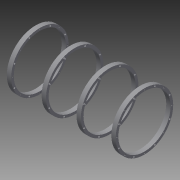
# Autodesk Inventor part: Part1
Saved by Autodesk Inventor 2015 (Build 190159000, 159)
## iProperties
Created: 2015-09-23
Part Number: Part1
Material: Generic
Document SubType Name: Modeling
Designer: Stefania
Density: 1 g/cm^3
Appearance: Default
Author: Stefania
Autodesk Inventor part; units mm, degrees
ref_plane "YZ Plane" through (0, 0, 0) normal (1, 0, 0) x (0, 1, 0)
ref_plane "XZ Plane" through (0, 0, 0) normal (0, 1, 0) x (-1, 0, 0)
ref_plane "Work Plane1" through (0, 0, 50.8) normal (0, 0, 1) x (1, 0, 0)
sketch "Sketch1" plane through (0, 0, 50.8) normal (0, 0, 1) x (1, 0, 0)
  circle A0 centre (0, 0) radius 76.2
  circle A1 centre (0, 0) radius 83.82
  dimension "d1" = 152.4
  dimension "d2" = 7.62
  constraints: 2 centre point, 1 coincident
  measures "d1" diameter of A0
  measures "d2" radial gap between concentric circles of A0 A1
extrude "Extrusion1" add sketch "Sketch1" along normal mid plane 12.7
pattern_linear "Rectangular Pattern1" count 3 spacing 101.6 along (0, 0, -1) count 2 spacing 101.6 along (0, 0, 1) of "Extrusion1"
sketch "Sketch2" plane through (0, 0, 158.75) normal (0, 0, 1) x (1, 0, 0)
  circle A0 centre (30.6185, 73.9196) radius 2.413
  circle A1 centre (-30.6185, 73.9196) radius 2.413
  circle A2 centre (-73.9196, 30.6185) radius 2.413
  circle A3 centre (-73.9196, -30.6185) radius 2.413
  circle A4 centre (-30.6185, -73.9196) radius 2.413
  circle A5 centre (30.6185, -73.9196) radius 2.413
  circle A6 centre (73.9196, -30.6185) radius 2.413
  circle A7 centre (73.9196, 30.6185) radius 2.413
  point P0 (0, 0)
  dimension "d16" = 4.826
  dimension "d19" = 360
  constraints: 8 centre point, 18 other
  measures "d16" diameter of A0
extrude "Extrusion2" cut sketch "Sketch2" against normal up to surface (12.7 mm away)
pattern_linear "Rectangular Pattern2" count 4 spacing 101.6 along (0, 0, -1) of "Extrusion2"
sketch "Sketch3" plane through (0, 0, 158.75) normal (0, 0, 1) x (1, 0, 0)
  circle A0 centre (0, 80.01) radius 1.7526
  circle A1 centre (-56.5756, 56.5756) radius 1.7526
  circle A2 centre (-80.01, 0) radius 1.7526
  circle A3 centre (-56.5756, -56.5756) radius 1.7526
  circle A4 centre (0, -80.01) radius 1.7526
  circle A5 centre (56.5756, -56.5756) radius 1.7526
  circle A6 centre (80.01, 0) radius 1.7526
  circle A7 centre (56.5756, 56.5756) radius 1.7526
  point P0 (0, 0)
  dimension "d26" = 3.5052
  dimension "d29" = 360
  constraints: 8 centre point, 18 other
  measures "d26" diameter of A0
extrude "Extrusion3" cut sketch "Sketch3" against normal up to surface (12.7 mm away)
pattern_linear "Rectangular Pattern4" count 2 spacing 304.8 along (0, 0, -1) of "Extrusion3"
thread "Thread1" size "6-32 UNC" class "2B" standard "ANSI Unified Screw Threads" full length
thread "Thread2" size "6-32 UNC" class "2B" standard "ANSI Unified Screw Threads" full length
thread "Thread3" size "6-32 UNC" class "2B" standard "ANSI Unified Screw Threads" full length
thread "Thread4" size "6-32 UNC" class "2B" standard "ANSI Unified Screw Threads" full length
thread "Thread5" size "6-32 UNC" class "2B" standard "ANSI Unified Screw Threads" full length
thread "Thread6" size "6-32 UNC" class "2B" standard "ANSI Unified Screw Threads" full length
thread "Thread7" size "6-32 UNC" class "2B" standard "ANSI Unified Screw Threads" full length
thread "Thread8" size "6-32 UNC" class "2B" standard "ANSI Unified Screw Threads" full length
thread "Thread9" size "6-32 UNC" class "2B" standard "ANSI Unified Screw Threads" full length
thread "Thread10" size "6-32 UNC" class "2B" standard "ANSI Unified Screw Threads" full length
thread "Thread11" size "6-32 UNC" class "2B" standard "ANSI Unified Screw Threads" full length
thread "Thread12" size "6-32 UNC" class "2B" standard "ANSI Unified Screw Threads" full length
thread "Thread13" size "6-32 UNC" class "2B" standard "ANSI Unified Screw Threads" full length
thread "Thread14" size "6-32 UNC" class "2B" standard "ANSI Unified Screw Threads" full length
thread "Thread15" size "6-32 UNC" class "2B" standard "ANSI Unified Screw Threads" full length
thread "Thread16" size "6-32 UNC" class "2B" standard "ANSI Unified Screw Threads" full length
thread "Thread17" size "6-32 UNC" class "2B" standard "ANSI Unified Screw Threads" full length
body "Solid1"
